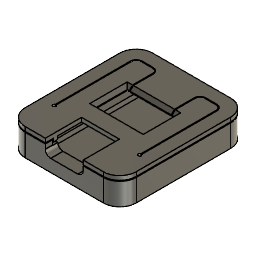
boardHolder (Autodesk Fusion 360 design; units mm, degrees)
Autodesk Fusion 360 part; units mm, degrees
note: some values were not read from the file. Chosen so that the rebuilt part matches the saved one: which face or edge a step refers to; a side. Set by a fixed rule: which sketch regions a step uses.
sketch "PCB Derived Dimensions" plane through (0, 0, 0) normal (0, 0, 1) x (1, 0, 0)
  line L0 (-10.5, -12.5) -> (10.5, -12.5)
  line L1 (10.5, -12.5) -> (10.5, 12.5)
  line L2 (10.5, 12.5) -> (-10.5, 12.5)
  line L3 (-10.5, 12.5) -> (-10.5, -12.5)
  line L4 (-10.5, -12.5) -> (10.5, 12.5) construction
  line L5 (10.5, -12.5) -> (-10.5, 12.5) construction
  line L6 (-7.5, 12.5) -> (-7.5, -12.5)
  line L7 (7.5, 12.5) -> (7.5, -12.5)
  line L8 (13.5, -15.5) -> (13.5, 15.5)
  line L9 (13.5, 15.5) -> (-13.5, 15.5)
  line L10 (-13.5, 15.5) -> (-13.5, -15.5)
  line L11 (-13.5, -15.5) -> (13.5, -15.5)
  line L12 (-5.7, 5.5) -> (5.7, 5.5)
  line L13 (5.7, 5.5) -> (5.7, -2)
  line L14 (5.7, -2) -> (-5.7, -2)
  line L15 (-5.7, -2) -> (-5.7, 5.5)
  line L16 (0, -2) -> (0, 0) construction
  line L17 (-4.6, -12.5) -> (-4.6, -15.5)
  line L18 (4.6, -12.5) -> (4.6, -15.5)
  dimension "d1" = 21
  dimension "d2" = 25
  dimension "d3" = 3
  dimension "d4" = 3
  dimension "d5" = 3
  dimension "d6" = 10.5
  dimension "d7" = 7
  dimension "d8" = 11.4
  dimension "d9" = 9.2
  constraint horizontal L0
  constraint perpendicular L0 L1
  constraint parallel L0 L2
  constraint parallel L1 L3
  constraint coincident L4 L16.end
  constraint coincident L5 L16.end
  constraint coincident L16.end origin
  constraint coincident L2 L6.start
  constraint coincident L0 L6.end
  constraint perpendicular L0 L6
  constraint coincident L2 L7.start
  constraint coincident L0 L7.end
  constraint perpendicular L0 L7
  constraint horizontal L12
  constraint vertical L13
  constraint horizontal L14
  constraint vertical L15
  constraint midpoint L14 L16.start
  constraint vertical L16
  constraint coincident L0 L17.start
  constraint coincident L11 L17.end
  constraint perpendicular L11 L17
  constraint coincident L0 L18.start
  constraint coincident L11 L18.end
  constraint perpendicular L11 L18
  constraint symmetric L16 L17 L18
  measures "d1" distance of L1.end L2.end
  measures "d2" distance of L0.end L1.end
  measures "d3" distance of L3 L6
  measures "d4" distance of L1 L7
  measures "d6" distance of L0 L14
  measures "d7" distance of L2 L12
  measures "d8" distance of L13 L15
  measures "d9" distance of L17 L18
sketch "Vertical Profile" plane through (0, 0, 0) normal (0, 1, 0) x (1, 0, 0)
  line L0 (-10.5, 0) -> (-7.5, 0)
  line L1 (-7.5, 0) -> (-7.5, 1.2)
  line L2 (-10.5, 0) -> (-10.5, -3.2)
  line L3 (-13.5, 0) -> (-13.5, -3.2)
  line L4 (-13.5, -3.2) -> (-10.5, -3.2)
  line L5 (-7.5, 1.2) -> (0, 1.2)
  line L6 (0, 1.2) -> (0, 0) construction
  line L7 (-13.5, -3.2) -> (-13.5, -3.4)
  point P0 (-7.5, 0)
  point P1 (-10.5, 0)
  point P2 (-13.5, 0)
  point P3 (-4.6, 0)
  point P4 (-10.5, -2.2)
  dimension "d10" = 1.2
  dimension "d11" = 3.2
  dimension "d25" = 0.2
  dimension "d26" = 1
  constraint coincident P1 L0.start
  constraint coincident P0 L0.end
  constraint perpendicular L0 L1
  constraint perpendicular L0 L2
  constraint coincident P2 L3.start
  constraint vertical L3
  constraint horizontal L4
  constraint perpendicular L1 L5
  constraint coincident L6.end origin
  constraint perpendicular L5 L6
  constraint perpendicular L4 L7
  constraint coincident L2 P4
  measures "d10" distance of P0 L1.end
  measures "d11" distance of P1 L2.end
  measures "d25" distance of L3.end L7.end
  measures "d26" distance of L2.end P4
extrude "Extrude1" add sketch "PCB Derived Dimensions" along normal up to surface (4.4 mm away) from surface at -1.2 contours L0 L1 L2 L3 L8 L9 L10 L11 L17 L18 | L0 L11 L17 L18 makes body 1
extrude "Extrude2" add sketch "PCB Derived Dimensions" against normal up to surface (1.2 mm away) contours L0 L2 L3 L6 | L0 L1 L2 L7 bodies 1
extrude "Extrude3" add sketch "PCB Derived Dimensions" against normal blind 1 from surface at -1.2 contours L0 L2 L3 L6 | L0 L1 L2 L3 L8 L9 L10 L11 L17 L18 | L0 L2 L6 L7 | L0 L11 L17 L18 | L0 L1 L2 L7 | L12 L13 L14 L15 bodies 1
extrude "Extrude4" cut sketch "PCB Derived Dimensions" against normal up to surface (2.4 mm away) from surface at 3.2 contours L0 L11 L17 L18 bodies 1
sketch "Top / Bottom Interface" plane through (0, 0, 3.2) normal (0, 0, 1) x (-1, 0, 0)
  line L0 (-4.6, 12.5) -> (-4.6, 15.5)
  line L1 (-4.6, 15.5) -> (-13.5, 15.5)
  line L2 (-13.5, 15.5) -> (-13.5, -15.5)
  line L3 (-13.5, -15.5) -> (13.5, -15.5)
  line L4 (13.5, -15.5) -> (13.5, 15.5)
  line L5 (4.6, 15.5) -> (4.6, 12.5)
  line L6 (4.6, 12.5) -> (10.5, 12.5)
  line L7 (10.5, 12.5) -> (10.5, -12.5)
  line L8 (10.5, -12.5) -> (-10.5, -12.5)
  line L9 (-10.5, -12.5) -> (-10.5, 12.5)
  line L10 (5.6, 13.5) -> (4.6, 13.5)
  line L11 (-5.6, 13.5) -> (-4.6, 13.5)
  line L12 (13.5, -15.5) -> (-13.5, -15.5)
  line L13 (-13.5, -15.5) -> (-13.5, 15.5)
  line L14 (-13.5, 15.5) -> (13.5, 15.5)
  line L15 (13.5, 15.5) -> (13.5, -15.5)
  line L16 (-10.5, 12.5) -> (-4.6, 12.5)
  line L17 (13.5, 15.5) -> (4.6, 15.5)
  line L18 (-11.5, -13.5) -> (-11.5, 13.5)
  line L19 (-11.5, 13.5) -> (-5.6, 13.5)
  line L20 (-5.6, 13.5) -> (-5.6, 14.5) construction
  line L21 (-5.6, 14.5) -> (-12.5, 14.5) construction
  line L22 (-12.5, 14.5) -> (-12.5, -14.5) construction
  line L23 (-12.5, -14.5) -> (12.5, -14.5) construction
  line L24 (12.5, -14.5) -> (12.5, 14.5) construction
  line L25 (12.5, 14.5) -> (5.6, 14.5)
  line L26 (5.6, 14.5) -> (5.6, 13.5) construction
  line L27 (5.6, 13.5) -> (11.5, 13.5)
  line L28 (11.5, 13.5) -> (11.5, -13.5)
  line L29 (11.5, -13.5) -> (-11.5, -13.5)
  dimension "d24" = -1
  constraint coincident L5 L10.end
  constraint perpendicular L5 L10
  constraint coincident L0 L11.end
  constraint perpendicular L0 L11
  constraint horizontal L12
  constraint vertical L13
  constraint horizontal L14
  constraint vertical L15
  constraint coincident L1.end L2.start
  constraint coincident L3.end L4.start
extrude "Extrude5" cut sketch "Top / Bottom Interface" against normal up to surface (1 mm away) contours L0 L5 L6 L7 L8 L9 L10 L11 L16 L18 L19 L27 L28 L29 bodies 1
move_face "OffsetFaces1" offset -0.2 6 faces at (-11.5, -4.5, 2.8667) (-3.8333, 13.5, 2.8667) (-11.1667, 4.1667, 2.2) (11.5, 4.5, 2.8667) (9.2, -13.5, 2.8667) (-6.9, -13.5, 2.8667) on bodies 1
extrude "Extrude6" add sketch "Top / Bottom Interface" along normal blind 1 from surface at 0.2 separate body makes body 2
extrude "Extrude7" cut sketch "PCB Derived Dimensions" along normal through all contours L12 L13 L14 L15 bodies 2
extrude "Extrude8" add sketch "Top / Bottom Interface" against normal blind 0.8 from surface at 0.2 contours L0 L5 L6 L7 L8 L9 L10 L11 L16 L18 L19 L27 L28 L29 bodies 2
sketch "Top Button Features" plane through (0, 0, 4.4) normal (0, 0, 1) x (-1, 0, 0)
  line L0 (-5.7, -5.5) -> (-5.7, 2)
  line L1 (-5.7, 2) -> (5.7, 2)
  line L2 (5.7, 2) -> (5.7, -5.5)
  line L3 (5.7, -5.5) -> (-5.7, -5.5)
  line L4 (13.5, 15.5) -> (-13.5, 15.5)
  line L5 (-13.5, 15.5) -> (-13.5, -15.5)
  line L6 (-13.5, -15.5) -> (13.5, -15.5)
  line L7 (13.5, -15.5) -> (13.5, 15.5)
  line L8 (10.5, -12.5) -> (6.9, -12.5) construction
  line L9 (-10.5, -12.5) -> (-6.9, -12.5) construction
  line L10 (10.5, -12.5) -> (10.5, 7.5)
  line L11 (10.5, -12.5) -> (5, -12.5)
  line L12 (5, -12.5) -> (5, -5.5)
  line L13 (5.7, -5.5) -> (-5.7, -5.5)
  line L14 (10.5, 7.5) -> (5.7, 7.5) construction
  line L15 (5.7, 7.5) -> (5.7, 2)
  line L16 (5.7, 2) -> (5.7, -5.5)
  line L17 (10.3, -12.3) -> (10.3, 7.5)
  line L18 (10.3, -12.3) -> (5.2, -12.3)
  line L19 (5.2, -12.3) -> (5.2, -5.5)
  line L20 (10.3, 7.5) -> (10.5, 7.5)
  line L21 (5, -12.5) -> (9, -12.5)
  line L22 (9, -12.5) -> (9, -8.5)
  line L23 (9, -8.5) -> (5, -8.5)
  line L24 (5, -8.5) -> (5, -12.5)
  line L25 (0, -5.5) -> (0, 0) construction
  line L26 (-10.3, -12.3) -> (-10.3, 7.5)
  line L27 (-10.5, -12.5) -> (-10.5, 7.5)
  line L28 (-10.3, 7.5) -> (-10.5, 7.5)
  line L29 (-10.5, -12.5) -> (-5, -12.5)
  line L30 (-10.3, -12.3) -> (-5.2, -12.3)
  line L31 (-5.2, -12.3) -> (-5.2, -5.5)
  line L32 (-5, -12.5) -> (-5, -5.5)
  line L33 (-9, -8.5) -> (-5, -8.5)
  line L34 (-9, -12.5) -> (-9, -8.5)
  line L35 (4.6, 15.5) -> (-4.6, 15.5)
  line L36 (-4.6, 15.5) -> (-4.6, 6.7)
  line L37 (-4.6, 6.7) -> (4.6, 6.7)
  line L38 (4.6, 6.7) -> (4.6, 15.5)
  point P0 (10.5, -12.5)
  point P1 (-10.5, -12.5)
  point P2 (4.6, 15.5)
  point P3 (-4.6, 15.5)
  point P4 (10.4, 7.5)
  point P5 (-10.4, 7.5)
  dimension "d37" = 3.6
  dimension "d38" = 20
  dimension "d39" = 5.5
  dimension "d41" = -0.2
  dimension "d42" = 4
  dimension "d43" = 4
  dimension "d45" = 8.8
  constraint coincident P0 L8.start
  constraint horizontal L8
  constraint coincident P1 L9.start
  constraint horizontal L9
  constraint equal L8 L9
  constraint perpendicular L8 L10
  constraint perpendicular L10 L11
  constraint perpendicular L11 L12
  constraint coincident L12.end L13
  constraint perpendicular L5 L14
  constraint coincident L1.end L2.start
  constraint vertical L15
  constraint perpendicular L10 L20
  constraint horizontal L21
  constraint vertical L22
  constraint horizontal L23
  constraint vertical L24
  constraint midpoint L13 L25.start
  constraint coincident L25.end origin
  constraint symmetric P0 L25 P1
  constraint symmetric L10.end L25 L27.end
  constraint symmetric L11.end L25 L29.end
  constraint symmetric L12.end L25 L32.end
  constraint symmetric L17.start L25 L26.start
  constraint symmetric L17.end L25 L26.end
  constraint symmetric L18.end L25 L30.end
  constraint symmetric L19.end L25 L31.end
  constraint symmetric L21.end L25 L34.start
  constraint symmetric L22.end L25 L33.start
  constraint symmetric L23.end L25 L33.end
  constraint coincident L13 L19.end
  constraint horizontal L35
  constraint vertical L36
  constraint horizontal L37
  constraint vertical L38
  constraint coincident P2 L35.start
  constraint coincident P3 L35.end
  constraint midpoint L20 P4
  constraint symmetric L25 P4 P5
  measures "d37" distance of P0 L8.end
  measures "d38" distance of P0 L10.end
  measures "d39" distance of P0 L11.end
  measures "d42" distance of L11.end L21.end
  measures "d43" distance of L11.end L23.end
  measures "d45" distance of P2 L37.end
sketch "Top Button Features Smoothed" plane through (0, 0, 4.4) normal (0, 0, 1) x (1, 0, 0)
  line L0 (-10.3, 12.3) -> (-5.2, 12.3) construction
  line L1 (-10.3, 12.3) -> (-10.3, -7.5) construction
  line L2 (-5.2, 12.3) -> (-5.2, 5.5) construction
  line L3 (5.2, 12.3) -> (5.2, 5.5) construction
  line L4 (10.3, 12.3) -> (5.2, 12.3) construction
  line L5 (10.3, 12.3) -> (10.3, -7.5) construction
  arc A0 (-9.1, 12.3) -> (-10.3, 11.1) centre (-9.1, 11.1) ccw
  line L6 (-7.75, 12.3) -> (-7.75, 10.3) construction
  arc A1 (-5.2, 11.1) -> (-6.4, 12.3) centre (-6.4, 11.1) ccw
  line L7 (-9.1, 12.3) -> (-6.4, 12.3)
  line L8 (-5.2, 11.1) -> (-5.2, 5.5)
  line L9 (-10.3, 11.1) -> (-10.3, -7.5)
  line L10 (0, 0) -> (0, 5.5)
  line L11 (-10.5, 11.1) -> (-10.5, -7.5)
  arc A2 (-9.1, 12.5) -> (-10.5, 11.1) centre (-9.1, 11.1) ccw
  line L12 (-9.1, 12.5) -> (-6.4, 12.5)
  arc A3 (-5, 11.1) -> (-6.4, 12.5) centre (-6.4, 11.1) ccw
  line L13 (-5, 11.1) -> (-5, 5.5)
  line L14 (-10.5, -7.5) -> (-10.3, -7.5)
  line L15 (-5.2, 5.5) -> (-5, 5.5)
  dimension "d54" = 1.2
  dimension "d55" = 2
  dimension "d56" = 0.2
  constraint coincident L1 A0.end
  constraint horizontal A0.centre A0.end
  constraint vertical A0.centre A0.start
  constraint coincident L0 A0.start
  constraint midpoint L0 L6.start
  constraint perpendicular L0 L6
  constraint symmetric A0.start L6 A1.end
  constraint symmetric A0.end L6 A1.start
  constraint symmetric A0 L6 A1
  constraint coincident L2.end L8.end
  constraint tangent A0 L9
  constraint coincident L10.start origin
  constraint parallel L5 L10
  constraint horizontal L2.end L10.end
  constraint horizontal L2.end L13.end
  constraint coincident L1.end L9.end
  constraint horizontal L1.end L11.end
  measures "d54" radius of A0
  measures "d55" distance of L6.start L6.end
chamfer "Chamfer1" distance 0.8 angle 45 4 edges at (0, 5.5, 4.4) (-5.7, 1.75, 4.4) (5.7, 1.75, 4.4) (0, -2, 4.4) on bodies 2
extrude "Extrude9" cut sketch "Top Button Features" along normal through all from surface at -1 contours L4 L35 L36 L37 L38 bodies 2
fillet "Fillet1" radius 4 8 edges at (-13.5, -15.5, 0.5) (13.5, -15.5, 0.5) (13.5, 15.5, 0.5) (-13.5, 15.5, 0.5) (-13.5, -15.5, 3.9) (13.5, -15.5, 3.9) (13.5, 15.5, 3.9) (-13.5, 15.5, 3.9) on bodies 1 2
extrude "Extrude11" cut sketch "Top Button Features Smoothed" against normal blind 1 bodies 2
hole "Hole1" at (-10.4, -7.5, 4.4) direction (0, 0, -1) diameter 0.8 depth 1 tip angle 180 bodies 2
mirror "Mirror1" about plane through (0, 0, 0) normal (1, 0, 0) of "Extrude11", "Hole1"
fillet "Fillet2" radius 1.3 2 edges at (4.6, -14, 0.8) (-4.6, -14, 0.8) on bodies 1
equation "d4 = d3"
equation "d45 = 5.8 mm + 3 mm"
named bodies: "bottom", "top"
